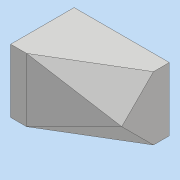
# Autodesk Inventor part: 16
Saved by Autodesk Inventor 2017 (Build 210142000, 142)
## iProperties
Part Number: 16
Material: 一般
Document SubType Name: Modeling
Designer: d8910
Density: 1 g/cm^3
Appearance: 預設
Author: d8910
Autodesk Inventor part; units mm, degrees
ref_plane "YZ Plane" through (0, 0, 0) normal (1, 0, 0) x (0, 1, 0)
ref_plane "XZ Plane" through (0, 0, 0) normal (0, 1, 0) x (-1, 0, 0)
sketch "草圖1" plane through (0, 0, 0) normal (0, 0, 1) x (1, 0, 0)
  line L0 (-15, 10) -> (15, 10)
  line L1 (15, 10) -> (15, -5)
  line L2 (-10, -10) -> (-15, -10)
  line L3 (-15, -10) -> (-15, 10)
  line L4 (-10, -10) -> (15, -5)
  point P0 (0, 0)
  point P1 (-15, 0)
  point P2 (0, 10)
  dimension "d0" = 30
  dimension "d1" = 20
  dimension "d2" = 5
  dimension "d3" = 15
  constraints: 10 end point, 2 horizontal alignment, 2 midpoint, 2 parallel, 1 horizontal, 1 perpendicular, 1 vertical alignment
  measures "d0" distance of L0.start L0.end
  measures "d1" distance of L2.end L0.start
  measures "d2" distance of L2.start L2.end
  measures "d3" distance of L0.end L1.end
extrude "擠出1" add sketch "草圖1" along normal blind 20
sketch "草圖2" plane through (0, 0, 20) normal (0, 0, 1) x (1, 0, 0)
  line L0 (-15, -10) -> (-10, -10) projected
  line L1 (-10, -10) -> (15, 5)
  line L2 (15, -5) -> (15, 10) projected
  point P0 (0, 0)
  dimension "d6" = 5
  constraints: 2 end point, 1 point on line
  measures "d6" distance of L2.end L1.end
sketch "草圖3" plane through (15, -5, 0) normal (1, 0, 0) x (0, 0, -1)
  line L0 (-20, 0) -> (-20, 15) construction
  line L1 (-20, 10) -> (-10, 0)
  line L2 (-20, -5) -> (-20, 10) construction
  point P0 (0, 5)
  dimension "d7" = 10
  constraints: 2 end point, 1 horizontal alignment
  measures "d7" distance of L1.end L0.start
sketch "草圖4" plane through (15, -5, 0) normal (0.1961161, -0.9805807, 0) x (0.9805807, 0.1961161, 0)
  line L0 (-25.4951, 20) -> (1.9612, 20) construction
  line L1 (1.9612, 20) -> (0, 10) construction
  line L2 (-25.4951, 20) -> (0, 10)
  point P0 (-13.7281, 0)
  constraints: 2 end point
ref_plane "工作平面1" through (15, 5, 20) normal (0.3905667, -0.6509446, 0.6509446) x (0, -0.7071068, -0.7071068)
sketch "草圖5" plane through (15, 5, 20) normal (0.3905667, -0.6509446, 0.6509446) x (0, -0.7071068, -0.7071068)
  line L0 (32.7788, -32.924) -> (-18.6727, -32.924)
  line L1 (-18.6727, -32.924) -> (-18.6727, 7.0938)
  line L2 (-18.6727, 7.0938) -> (32.7788, 7.0938)
  line L3 (32.7788, 7.0938) -> (32.7788, -32.924)
  point P0 (17.6777, -9.666)
  constraints: 8 end point, 2 parallel, 1 horizontal, 1 perpendicular
extrude "擠出2" cut sketch "草圖5" along normal through all
sketch "草圖6" plane through (15, -5, 0) normal (1, 0, 0) x (0, 0, -1)
  line L0 (0, 0) -> (-10, 0) projected
  line L1 (-10, 0) -> (-10, 25.1202)
  point P0 (0, 5)
  constraints: 2 end point, 1 vertical
surface extrude "擠出表面1" sketch "草圖6" against normal blind 63.25 shown no curves L0 L1
mirror "鏡射1" about plane through (15, -5, 10) normal (0, 0, 1) of "擠出2"
